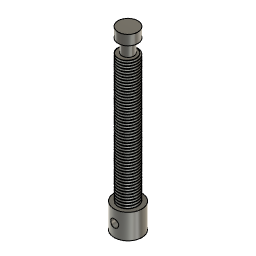
Part IV - Screw v1 (Autodesk Fusion 360 design; units mm, degrees)
Autodesk Fusion 360 part; units mm, degrees
sketch "Sketch1" plane through (0, 0, 0) normal (0, 0, 1) x (1, 0, 0)
  circle A0 centre (0, 0) radius 14
  dimension "d1" = 28
  constraint coincident A0.centre origin
  measures "d1" diameter of A0
extrude "Extrude1" add sketch "Sketch1" along normal blind 25
sketch "Sketch2" plane through (0, 0, 25) normal (0, 0, 1) x (-1, 0, 0)
  circle A0 centre (0, 0) radius 14
  circle A1 centre (0, 0) radius 10
  dimension "d4" = 20
  constraint coincident A0.centre A1.centre
  measures "d4" diameter of A1
extrude "Extrude2" add sketch "Sketch2" along normal blind 130 contours A1
sketch "Sketch3" plane through (0, 0, 155) normal (0, 0, 1) x (-1, 0, 0)
  circle A0 centre (0, 0) radius 10
  circle A1 centre (0, 0) radius 6
  dimension "d7" = 12
  constraint coincident A0.centre A1.centre
  measures "d7" diameter of A1
extrude "Extrude3" add sketch "Sketch3" along normal blind 13 contours A1
sketch "Sketch4" plane through (0, 0, 168) normal (0, 0, 1) x (-1, 0, 0)
  circle A0 centre (0, 0) radius 6
  circle A1 centre (0, 0) radius 10
  dimension "d10" = 20
  constraint coincident A0.centre A1.centre
  measures "d10" diameter of A1
extrude "Extrude4" add sketch "Sketch4" along normal blind 10 contours A0 | A1
sketch "Sketch5" plane through (0, 0, 0) normal (0, 1, 0) x (1, 0, 0)
  line L0 (-14, -25) -> (14, -25)
  line L1 (-14, -25) -> (14, -25)
  line L2 (-14, 0) -> (14, 0)
  circle A0 centre (0, -12.5) radius 4
  dimension "d13" = 8
  dimension "d14" = 14
  dimension "d15" = 12.5
  measures "d13" diameter of A0
  measures "d14" horizontal distance of L0.end A0.centre
  measures "d15" distance of L2 A0.centre
extrude "Extrude5" cut sketch "Sketch5" along normal through all and the other way through all
thread "Thread1" "ISO Metric profile 20.0 M20x2.5 6g" major diameter 19.7905 minor diameter 16.938 pitch 2.5 angle 60 modelled right hand crest width 0.36 on face at (-9.9503, 0.9957, 68.3333) crest through (-9.8953, 0, 24.375)
